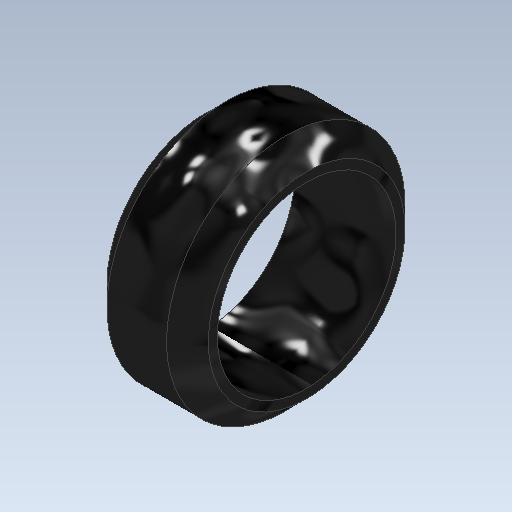
# Autodesk Inventor part: pom wheel
Saved by Autodesk Inventor 2020 (Build 240168000, 168)
## iProperties
Created: 2021-03-19
Part Number: pom wheel
Material: Acetal Resin, Black
Document SubType Name: Modeling
Designer: AOB
Mass: 2.43059 g
Surface Area: 15.4472 cm^2
Volume: 1.70568 cm^3
Density: 1.425 g/cm^3
Appearance: Black
Author: AOB
Autodesk Inventor part; units mm, degrees
ref_plane "YZ Plane" through (0, 0, 0) normal (1, 0, 0) x (0, 1, 0)
ref_plane "XZ Plane" through (0, 0, 0) normal (0, 1, 0) x (-1, 0, 0)
sketch "Sketch1" plane through (0, 0, 0) normal (0, 0, 1) x (1, 0, 0)
  line L0 (2.1, 0) -> (8.1, 0)
  line L1 (10.2, -2.1) -> (10.2, -9.55)
  line L2 (10.2, -12) -> (0, -12)
  line L3 (0, -9.55) -> (0, -2.1)
  line L4 (2.1, 0) -> (0, -2.1)
  line L5 (8.1, 0) -> (10.2, -2.1)
  line L6 (0, -9.55) -> (10.2, -9.55)
  line L7 (0, -3) -> (10.2, -3)
  point P0 (0, 0)
  point P1 (10.2, 0)
  dimension "d0" = 10.2
  dimension "d1" = 12
  dimension "d2" = 2.1
  dimension "d3" = 45
  dimension "d4" = 2.1
  dimension "d5" = 45
  dimension "d6" = 2.45
  dimension "d7" = 9
  constraints: 16 end point, 6 point on line, 3 perpendicular, 2 parallel, 1 horizontal
  measures "d0" distance of point (0, 0) point (10.2, 0)
  measures "d1" distance of point (10.2, 0) L2.start
  measures "d2" distance of L0.start point (0, 0)
  measures "d3" angle of L0 L4
  measures "d4" distance of L0.end point (10.2, 0)
  measures "d5" angle of L0 L5
  measures "d6" distance between parallel lines of L2 L6
  measures "d7" distance between parallel lines of L2 L7
revolve "Revolution1" add sketch "Sketch1" angle 360 about axis through (10.2, -12, 0) along (-1, 0, 0) contours L0 L5 L1 L7 L3 L4
ref_plane "Work Plane1" through (5.1, -12, 0) normal (-1, 0, 0) x (0, 0, 1)
equation "\"d4\" = d2"
equation "\"d5\" = d3"
body "Solid1"
